Window Sill Helper (Autodesk Fusion 360 design; units mm, degrees)
Autodesk Fusion 360 part; units mm, degrees
sketch "Sketch1" plane through (0, 0, 0) normal (0, 0, 1) x (1, 0, 0)
  circle A0 centre (0, 0) radius 6
  circle A1 centre (0, 0) radius 7.5
  circle A2 centre (0, 0) radius 5.15
  dimension "d1" = 12
  dimension "d2" = 15
  dimension "d3" = 10.3
  constraint coincident A0.centre A1.centre
  constraint concentric A0 A1
  measures "d1" diameter of A0
  measures "d2" diameter of A1
  measures "d3" diameter of A2
extrude "Extrude1" add sketch "Sketch1" along normal blind 4.2 contours A0 | A1
chamfer "Chamfer1" distance 0.8 distance2 4.2 1 edges at (-4.8015, 1.8623, 4.2) measured on face at (6.6696, -0.6285, 4.2)
extrude "Extrude2" add sketch "Sketch1" against normal blind 3 contours A0 | A1 | A2
